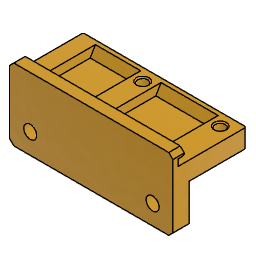
cnc3018_EndstopXY v5 (Autodesk Fusion 360 design; units mm, degrees)
Autodesk Fusion 360 part; units mm, degrees
sketch "Skizze1" plane through (0, 0, 0) normal (0, 0, 1) x (1, 0, 0)
  line L0 (0, 0) -> (40, 0)
  line L1 (40, 0) -> (40, 18)
  line L2 (40, 18) -> (0, 18)
  line L3 (0, 18) -> (0, 0)
  circle A0 centre (36.6, 15) radius 1.25
  circle A1 centre (17.6, 15) radius 1.25
  line L4 (36.6, 15) -> (17.6, 15) construction
  line L5 (0, 0) -> (40, 0)
  line L6 (40, 0) -> (40, 4)
  line L7 (40, 4) -> (0, 4)
  line L8 (0, 4) -> (0, 0)
  line L9 (0, 18) -> (4, 18)
  line L10 (4, 18) -> (4, 0)
  line L11 (4, 0) -> (0, 0)
  line L12 (0, 0) -> (0, 18)
  line L13 (17.6, 18) -> (17.6, 4) construction
  line L14 (36.6, 18) -> (36.6, 4) construction
  line L15 (15.1, 18) -> (15.1, 4)
  line L16 (34.1, 18) -> (34.1, 4)
  line L17 (20.1, 18) -> (20.1, 4)
  line L18 (4, 17) -> (40, 17)
  dimension "d1" = 40
  dimension "d2" = 18
  dimension "d3" = 19
  dimension "d4" = 2.5
  dimension "d5" = 3
  dimension "d6" = 3.4
  dimension "d7" = 4
  dimension "d8" = 2.5
  dimension "d9" = 5
  dimension "d17" = 1
  dimension "d36" = 4
  constraint horizontal L0
  constraint vertical L1
  constraint horizontal L2
  constraint vertical L3
  constraint coincident L0.start L3.end
  constraint coincident A0.centre L4.start
  constraint coincident A1.centre L4.end
  constraint parallel L2 L4
  constraint equal A0 A1
  constraint horizontal L5
  constraint vertical L6
  constraint horizontal L7
  constraint vertical L8
  constraint coincident L1 L6.end
  constraint horizontal L9
  constraint vertical L10
  constraint horizontal L11
  constraint vertical L12
  constraint coincident L0 L10.end
  constraint coincident L2 L13.start
  constraint coincident L7 L13.end
  constraint perpendicular L7 L13
  constraint coincident A1.centre L13
  constraint coincident L2 L14.start
  constraint coincident L7 L14.end
  constraint perpendicular L7 L14
  constraint coincident A0.centre L14
  constraint coincident L2 L15.start
  constraint coincident L7 L15.end
  constraint perpendicular L7 L15
  constraint coincident L2 L16.start
  constraint coincident L7 L16.end
  constraint perpendicular L7 L16
  constraint symmetric L13 L15.start L17.start
  constraint symmetric L13 L15.end L17.end
  constraint coincident L10 L18.start
  constraint coincident L1 L18.end
  constraint perpendicular L1 L18
  measures "d1" distance of L0.start L0.end
  measures "d2" distance of L0.start L2.end
  measures "d3" distance of A0.centre A1.centre
  measures "d4" diameter of A1
  measures "d5" distance of L2 L4
  measures "d6" distance of L1 A0.centre
  measures "d7" distance of L5 L7
  measures "d8" distance of L14 L16
  measures "d9" distance of L15 L17
  measures "d17" distance of L2 L18
  measures "d36" distance of L3 L10
extrude "Extrusion1" add sketch "Skizze1" along normal blind 4.5
extrude "Extrusion2" cut sketch "Skizze1" against normal blind 2.2 from surface at 4.5 contours L7 L10 L15 L18 | L7 L16 L17 L18
extrude "Extrusion3" add sketch "Skizze1" against normal blind 10 contours L0 L3 L5 L7 L8 L10 L11 L12 | L0 L1 L5 L6 L7 L10
sketch "Skizze2" plane through (0, 0, 0) normal (0, -1, 0) x (1, 0, 0)
  line L0 (40, -10) -> (40, 4.5)
  line L1 (40, 4.5) -> (0, 4.5)
  line L2 (0, 4.5) -> (0, -10)
  line L3 (0, -10) -> (40, -10)
  line L4 (20, -10) -> (20.1, 4.5) construction
  line L5 (40, 0) -> (0, 0) construction
  circle A0 centre (5.0338, -5) radius 1.6
  circle A1 centre (35.0338, -5.2069) radius 1.6
  point P0 (20.1, 4.5)
  dimension "d18" = 3.2
  dimension "d19" = 5
  dimension "d35" = 30
  constraint midpoint L3 L4.start
  constraint coincident P0 L4.end
  constraint symmetric L4 A0 A1
  measures "d18" diameter of A0
  measures "d19" distance of L5 A0.centre
  measures "d35" horizontal distance of A0.centre A1.centre
extrude "Extrusion4" cut sketch "Skizze2" against normal through all contours A0 | A1
chamfer "Fase1" distance 2.2 angle 30 2 edges at (9.55, 17, 2.3) (27.1, 17, 2.3) measured on face at (7.7, 17, 3.7667) measured on face at (24.7667, 17, 3.7667)
sketch "Skizze3" plane through (40, 0, 0) normal (1, 0, 0) x (0, 1, 0)
  line L0 (4, 0) -> (18, 0)
  line L1 (18, 0) -> (18, 4.5)
  line L2 (18, 4.5) -> (0, 4.5)
  line L3 (0, 4.5) -> (0, -10)
  line L4 (0, -10) -> (4, -10)
  line L5 (4, -10) -> (4, 0)
  line L6 (0, 4.5) -> (0, 7.6)
  line L7 (0, 7.6) -> (2.8, 7.6)
  line L8 (2.8, 7.6) -> (2.8, 6.1)
  line L9 (2.8, 6.1) -> (1.3, 6.1)
  line L10 (1.3, 6.1) -> (1.3, 4.5)
  point P0 (18, 4.5)
  dimension "d23" = 16.7
  dimension "d24" = 1.6
  dimension "d25" = 1.5
  dimension "d26" = 1.5
  constraint coincident L2.end L3.start
  constraint perpendicular L2 L6
  constraint perpendicular L6 L7
  constraint perpendicular L7 L8
  constraint perpendicular L8 L9
  constraint coincident L2 L10.end
  constraint perpendicular L2 L10
  measures "d23" distance of L10 P0
  measures "d24" distance of L2 L9
  measures "d25" distance of L7 L9
  measures "d26" distance of L8.end L9.end
extrude "Extrusion5" add sketch "Skizze3" against normal blind 40 contours L2 L6 L7 L8 L9 L10
chamfer "Fase2" distance 1 angle 45 4 edges at (0, 2, -10) (40, 2, -10) (40, 1.4, 7.6) (0, 1.4, 7.6) measured on face at (13.3333, 2.6667, -10) measured on face at (13.3333, 2.6667, -10) measured on face at (26.6667, 0.9333, 7.6) measured on face at (0, 7.7667, 3)
chamfer "Fase2" distance 0.3 angle 45 3 edges at (20, 2.8, 6.1) (40, 18, 2.25) (0, 18, 2.25) measured on face at (26.6667, 2.8, 7.1) measured on face at (40, 7.7667, 3) measured on face at (26.6667, 18, 1.5)
chamfer "Fase2" distance 0.3 angle 45 4 edges at (16.4346, 15.452, 4.5) (35.4346, 15.452, 4.5) (35.4346, 15.452, 0) (16.4346, 15.452, 0) measured on face at (37.0522, 6.3788, 4.5) measured on face at (37.0522, 6.3788, 4.5) measured on face at (37.8484, 14.9377, 3) measured on face at (18.8484, 14.9377, 3)
